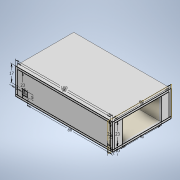
# Autodesk Inventor part: Деталь2
Saved by Autodesk Inventor 2020 (Build 240168000, 168)
## iProperties
Created: 2023-05-15
Part Number: Деталь2
Material: Типовые
Document SubType Name: Modeling
Designer: kikim
Density: 1 g/cm^3
Appearance: По умолчанию
Author: kikim
Autodesk Inventor part; units mm, degrees
ref_plane "XZ Plane" through (0, 0, 0) normal (0, 1, 0) x (-1, 0, 0)
ref_plane "XY Plane" through (0, 0, 0) normal (0, 0, 1) x (1, 0, 0)
sketch "Эскиз1" plane through (0, 0, 0) normal (1, 0, 0) x (0, 1, 0)
  line L0 (0, 0) -> (25, 0)
  line L1 (25, 0) -> (25, -60)
  line L2 (25, -60) -> (0, -60)
  line L3 (0, -60) -> (0, 0)
  line L4 (0, 0) -> (0, -2)
  line L5 (0, -2) -> (23, -2)
  line L6 (23, -2) -> (23, -58)
  line L7 (23, -58) -> (0, -58)
  line L8 (0, 0) -> (0, -10)
  line L9 (0, -10) -> (23, -10)
  line L10 (0, -10) -> (0, -50)
  line L11 (0, -50) -> (23, -50)
  line L12 (0, 0) -> (-2, 0)
  line L13 (-2, 0) -> (-2, -60)
  line L14 (-2, -60) -> (0, -60)
  line L15 (0, -10) -> (0, -50)
  dimension "d0" = 25
  dimension "d1" = 60
  dimension "d2" = 2
  dimension "d3" = 23
  dimension "d4" = 56
  dimension "d5" = 10
  dimension "d6" = 40
  dimension "d26" = 2
  constraints: 32 end point, 9 perpendicular, 6 point on line, 2 horizontal, 1 collinear, 1 parallel
  measures "d0" distance of L0.start L0.end
  measures "d1" distance of L0.end L1.end
  measures "d2" distance of L0.start L4.end
  measures "d3" distance of L4.end L5.end
  measures "d4" distance of L5.end L6.end
  measures "d5" distance of L0.start L8.end
  measures "d6" distance of L8.end L10.end
  measures "d26" distance of L0.start L12.end
sketch "Эскиз2" plane through (0, 0, 0) normal (0, 0, 1) x (1, 0, 0)
  line L0 (0, 0) -> (0, 25)
  line L1 (0, 25) -> (-100, 25)
  line L2 (-100, 25) -> (-100, 0)
  line L3 (-100, 0) -> (0, 0)
  line L4 (-100, 0) -> (-98, 0)
  line L5 (-98, 0) -> (-98, 23)
  line L6 (-98, 23) -> (-2, 23)
  line L7 (-2, 23) -> (-2, 0)
  line L8 (-98, 0) -> (-93, 0)
  line L9 (-93, 3) -> (-88, 3)
  line L10 (-88, 3) -> (-88, 8)
  line L11 (-88, 8) -> (-93, 8)
  line L12 (-93, 8) -> (-93, 3)
  line L13 (0, 0) -> (0, -2)
  line L14 (0, -2) -> (-100, -2)
  line L15 (-100, -2) -> (-100, 0)
  line L16 (-98, 0) -> (-2, 0)
  dimension "d7" = 25
  dimension "d8" = 100
  dimension "d9" = 2
  dimension "d10" = 23
  dimension "d11" = 96
  dimension "d13" = 3
  dimension "d14" = 5
  dimension "d15" = 5
  dimension "d16" = 88
  dimension "d17" = 17
  dimension "d27" = 2
  constraints: 34 end point, 11 perpendicular, 3 point on line, 2 parallel, 2 vertical
  measures "d7" distance of L0.start L0.end
  measures "d8" distance of L0.end L1.end
  measures "d9" distance of L2.end L4.end
  measures "d10" distance of L4.end L5.end
  measures "d11" distance of L5.end L6.end
  measures "d13" distance of L8.end L9.start
  measures "d14" distance of L9.start L9.end
  measures "d15" distance of L9.end L10.end
  measures "d16" distance between parallel lines of L10 L0
  measures "d17" distance between parallel lines of L11 L1
  measures "d27" distance of L0.start L13.end
ref_plane "РабПлоскость3" through (-2, 0, 0) normal (1, 0, 0) x (0, 1, 0)
sketch "Эскиз3" plane through (-2, 0, 0) normal (1, 0, 0) x (0, 1, 0)
  line L0 (0, 0) -> (0, -2)
  line L1 (0, -2) -> (23, -2)
  line L2 (23, -2) -> (23, -58)
  line L3 (23, -58) -> (0, -58)
  line L4 (0, -58) -> (0, -50)
  line L5 (0, -50) -> (23, -50)
  line L6 (23, -50) -> (23, -10)
  line L7 (23, -10) -> (0, -10)
  line L8 (0, -10) -> (0, -2)
  line L9 (0, -50) -> (0, -58)
  dimension "d30" = 2
  dimension "d31" = 23
  dimension "d32" = 56
  dimension "d33" = 8
  dimension "d34" = 40
  constraints: 20 end point, 6 perpendicular, 5 point on line, 1 collinear, 1 vertical
  measures "d30" distance of L0.start L0.end
  measures "d31" distance of L0.end L1.end
  measures "d32" distance of L1.end L2.end
  measures "d33" distance of L3.end L4.end
  measures "d34" distance of L5.end L6.end
extrude "Выдавливание5" add sketch "Эскиз2" against normal blind 60 contours L3 L7 L6 L5 L2 L1 L0 | L3 L5 L6 L7
extrude "Выдавливание6" add sketch "Эскиз2" against normal blind 60 contours L13 L14 L15 L3
extrude "Выдавливание7" cut sketch "Эскиз1" against normal blind 98 contours L9 L6 L11 L3
extrude "Выдавливание8" add sketch "Эскиз3" against normal blind 98
